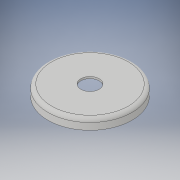
# Autodesk Inventor part: DireccionBase
Saved by Autodesk Inventor 2019 (Build 230136000, 136)
## iProperties
Created: 2020-04-23
Part Number: DireccionBase
Material: Generic
Document SubType Name: Modeling
Designer: Sergio
Density: 1 g/cm^3
Appearance: Default
Author: Sergio
Autodesk Inventor part; units mm, degrees
ref_plane "YZ Plane" through (0, 0, 0) normal (1, 0, 0) x (0, 1, 0)
ref_plane "XZ Plane" through (0, 0, 0) normal (0, 1, 0) x (-1, 0, 0)
ref_plane "XY Plane" through (0, 0, 0) normal (0, 0, 1) x (1, 0, 0)
sketch "Sketch1" plane through (0, 0, 0) normal (0, 1, 0) x (-1, 0, 0)
  circle A0 centre (0, 0) radius 66.5
  circle A1 centre (0, 0) radius 15
  dimension "d0" = 133
  dimension "d3" = 30
  constraints: 2 centre point, 2 coincident
  measures "d0" diameter of A0
  measures "d3" diameter of A1
extrude "Extrusion2" add sketch "Sketch1" along normal blind 3
sketch "Sketch3" plane through (0, 3, 0) normal (0, 1, 0) x (1, 0, 0)
  circle A0 centre (0, 0) radius 66.5
  circle A1 centre (0, 0) radius 68.5
  dimension "d6" = 133
  dimension "d7" = 137
  constraints: 2 centre point, 2 coincident
  measures "d6" diameter of A0
  measures "d7" diameter of A1
extrude "Extrusion3" add sketch "Sketch3" against normal blind 17
sketch "Sketch4" plane through (0, 0, 0) normal (0, -1, 0) x (1, 0, 0)
  circle A0 centre (0, 0) radius 15
  circle A1 centre (0, 0) radius 39
  line L0 (10.6103, -10.6029) -> (27.5808, -27.5735)
  line L1 (39, 0) -> (15, 0)
  circle A2 centre (0, 0) radius 15 projected
  line L2 (27.7885, -27.3642) -> (10.8166, -10.3923)
  dimension "d10" = 30
  dimension "d11" = 24
  constraints: 6 end point, 4 point on circle, 3 coincident, 2 centre point, 1 horizontal, 1 other
  measures "d10" diameter of A0
  measures "d11" radial gap between concentric circles of A1 A0
extrude "Extrusion4" cut sketch "Sketch4" against normal blind 1.5 contours L1 A1 L2 A0 | A0 L2 A1 L0
mirror "Mirror1" about plane through (0, 0, 0) normal (0, 0, 1) of "Extrusion4"
fillet "Fillet1" radius 6 1 edges at (-68.5, 3, 0)
fillet "Fillet2" radius 2 1 edges at (-66.5, 0, 0)
body "Solid2"
